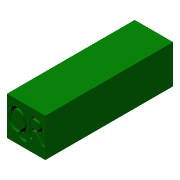
# Autodesk Inventor part: Container 2 2 5 QR color 2
Saved by Autodesk Inventor 2015 (Build 190159000, 159)
## iProperties
Created: 2015-03-07
Part Number: Container 2 2 5 QR color 2
Material: Generic
Document SubType Name: Modeling
Designer: Vukica
Density: 1 g/cm^3
Appearance: Dark Green
Author: Vukica
Autodesk Inventor part; units mm, degrees
ref_plane "YZ Plane" through (0, 0, 0) normal (1, 0, 0) x (0, 1, 0)
ref_plane "XZ Plane" through (0, 0, 0) normal (0, 1, 0) x (-1, 0, 0)
ref_plane "XY Plane" through (0, 0, 0) normal (0, 0, 1) x (1, 0, 0)
sketch "Sketch1" plane through (0, 0, 0) normal (0, 0, 1) x (1, 0, 0)
  line L0 (0, 0) -> (38.1, 0)
  line L1 (38.1, 0) -> (38.1, 38.1)
  line L2 (38.1, 38.1) -> (0, 38.1)
  line L3 (0, 38.1) -> (0, 0)
  dimension "d0" = 38.1
  dimension "d1" = 38.1
  constraints: 8 end point, 2 parallel, 1 horizontal, 1 perpendicular
  measures "d0" distance of L1.end L2.end
  measures "d1" distance of L2.end L0.start
extrude "Extrusion1" add sketch "Sketch1" along normal blind 127
sketch "Sketch2" plane through (0, 0, 127) normal (0, 0, 1) x (1, 0, 0)
  line L0 (0.4411, 31.4991) -> (46.8362, 31.4991) construction
  line L1 (46.8362, 31.4991) -> (46.8362, -1.1257) construction
  line L2 (46.8362, -1.1257) -> (0.4411, -1.1257) construction
  line L3 (0.4411, -1.1257) -> (0.4411, 31.4991) construction
  spline S0 degree 2 poles (19.3779, 5.7779) (18.6369, 5.5968) (17.0231, 5.3992) (16.2163, 5.3992) knots 0 0 0 1 2 2 2
  spline S1 degree 2 poles (16.2163, 5.3992) (13.9274, 5.3992) (11.0786, 7.9516) (10.9469, 10.3228) knots 0 0 0 1 2 2 2
  spline S2 degree 2 poles (10.9469, 10.3228) (10.7658, 10.3228) (10.4529, 10.3228) (10.3211, 10.3228) knots 0 0 0 1 2 2 2
  spline S3 degree 2 poles (10.3211, 10.3228) (8.2628, 10.3228) (4.953, 11.7225) (3.7674, 13.0892) knots 0 0 0 1 2 2 2
  spline S4 degree 2 poles (3.7674, 13.0892) (2.5982, 14.4395) (1.3468, 18.3915) (1.3468, 20.8944) knots 0 0 0 1 2 2 2
  spline S5 degree 2 poles (1.3468, 20.8944) (1.3468, 23.4633) (2.6147, 27.3494) (3.7838, 28.7326) knots 0 0 0 1 2 2 2
  spline S6 degree 2 poles (3.7838, 28.7326) (4.9694, 30.0994) (8.2793, 31.4991) (10.3211, 31.4991) knots 0 0 0 1 2 2 2
  spline S7 degree 2 poles (10.3211, 31.4991) (12.396, 31.4991) (15.7223, 30.05) (16.8749, 28.7326) knots 0 0 0 1 2 2 2
  spline S8 degree 2 poles (16.8749, 28.7326) (18.0276, 27.3988) (19.312, 23.4303) (19.312, 20.8944) knots 0 0 0 1 2 2 2
  spline S9 degree 2 poles (19.312, 20.8944) (19.312, 16.9424) (16.2327, 11.8048) (13.5486, 10.8991) knots 0 0 0 1 2 2 2
  spline S10 degree 2 poles (13.5486, 10.8991) (13.6145, 10.1416) (14.0097, 8.9231) (14.3226, 8.5773) knots 0 0 0 1 2 2 2
  spline S11 degree 2 poles (14.3226, 8.5773) (14.7013, 8.1492) (15.7387, 7.754) (16.6609, 7.754) knots 0 0 0 1 2 2 2
  spline S12 degree 2 poles (16.6609, 7.754) (17.2043, 7.754) (18.6863, 8.0998) (19.0156, 8.2315) knots 0 0 0 1 2 2 2
  line L4 (19.0156, 8.2315) -> (19.3779, 8.2315)
  line L5 (19.3779, 8.2315) -> (19.3779, 5.7779)
  spline S13 degree 2 poles (16.4962, 20.8944) (16.4962, 22.9199) (15.6234, 26.0321) (14.833, 27.053) knots 0 0 0 1 2 2 2
  spline S14 degree 2 poles (14.833, 27.053) (14.0262, 28.1069) (11.7538, 29.1608) (10.3376, 29.1608) knots 0 0 0 1 2 2 2
  spline S15 degree 2 poles (10.3376, 29.1608) (8.8721, 29.1608) (6.6655, 28.1398) (5.8257, 27.053) knots 0 0 0 1 2 2 2
  spline S16 degree 2 poles (5.8257, 27.053) (5.0188, 26.0156) (4.1626, 22.8705) (4.1626, 20.8944) knots 0 0 0 1 2 2 2
  spline S17 degree 2 poles (4.1626, 20.8944) (4.1626, 16.893) (7.5218, 12.6281) (10.3376, 12.6281) knots 0 0 0 1 2 2 2
  spline S18 degree 2 poles (10.3376, 12.6281) (13.1534, 12.6281) (16.4962, 16.893) (16.4962, 20.8944) knots 0 0 0 1 2 2 2
  line L6 (38.0018, 10.7509) -> (34.4944, 10.7509)
  line L7 (34.4944, 10.7509) -> (28.0723, 18.8361)
  line L8 (28.0723, 18.8361) -> (24.9766, 18.8361)
  line L9 (24.9766, 18.8361) -> (24.9766, 10.7509)
  line L10 (24.9766, 10.7509) -> (22.276, 10.7509)
  line L11 (22.276, 10.7509) -> (22.276, 31.0709)
  line L12 (22.276, 31.0709) -> (27.5125, 31.0709)
  spline S19 degree 2 poles (27.5125, 31.0709) (29.2579, 31.0709) (31.6127, 30.6922) (32.683, 30.0006) knots 0 0 0 1 2 2 2
  spline S20 degree 2 poles (32.683, 30.0006) (33.7534, 29.309) (34.9884, 27.1518) (34.9884, 25.5545) knots 0 0 0 1 2 2 2
  spline S21 degree 2 poles (34.9884, 25.5545) (34.9884, 23.3315) (32.716, 20.3181) (30.7729, 19.5936) knots 0 0 0 1 2 2 2
  line L13 (30.7729, 19.5936) -> (38.0018, 10.7509)
  spline S22 degree 2 poles (32.1726, 25.3405) (32.1726, 26.2297) (31.5468, 27.5964) (30.8882, 28.041) knots 0 0 0 1 2 2 2
  spline S23 degree 2 poles (30.8882, 28.041) (30.3118, 28.4198) (28.7804, 28.7326) (27.6607, 28.7326) knots 0 0 0 1 2 2 2
  line L14 (27.6607, 28.7326) -> (24.9766, 28.7326)
  line L15 (24.9766, 28.7326) -> (24.9766, 21.092)
  line L16 (24.9766, 21.092) -> (27.3478, 21.092)
  spline S24 degree 2 poles (27.3478, 21.092) (28.5169, 21.092) (30.3777, 21.5037) (31.0199, 22.1459) knots 0 0 0 1 2 2 2
  spline S25 degree 2 poles (31.0199, 22.1459) (31.6127, 22.7058) (32.1726, 24.2866) (32.1726, 25.3405) knots 0 0 0 1 2 2 2
  point P0 (0, 0)
  constraints: 2 other
extrude "Extrusion2" cut sketch "Sketch2" against normal blind 2.54
body "Solid1"
